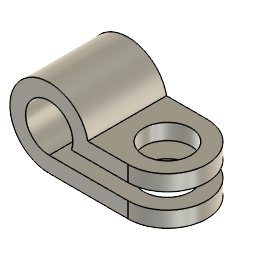
Cable Clip (Autodesk Fusion 360 design; units mm, degrees)
part number: 2025-09-15-17-10-41-254
part number: 2025-09-15-17-13-02-400
Autodesk Fusion 360 part; units mm, degrees
sketch "Sketch1" plane through (0, 0, 0) normal (0, 0, 1) x (1, 0, 0) in component "3mm Cable Clip"
sketch "Sketch2" plane through (0, 0, 0) normal (0, 1, 0) x (1, 0, 0) in component "3mm Cable Clip"
  line L0 (0, 3) -> (15, 3)
  line L1 (0, 0) -> (0, 3) construction
  line L2 (2.8284, 1) -> (15, 1)
  arc A0 (0, 3) -> (2.8284, 1) centre (0, 0) ccw
  dimension "d2" = 6
  dimension "d3" = 15
  dimension "d5" = 2
  constraint coincident L1.start A0.centre
  constraint horizontal L0
  constraint perpendicular L0 L1
  constraint horizontal L2
  constraint vertical L0.end L2.end
  measures "d2" diameter of A0
  measures "d3" distance of L0.start L0.end
  measures "d5" distance of L0 L2
surface "Extrude1" add extruded along (0, 1, 0) between 0 and 10 path "Sketch2" along L0 A0 L2 makes body 1 in component "3mm Cable Clip"
thicken "Thicken1" add thickness 2 3 faces at (-2.5433, 6.6667, 1.5912) (5, 3.3333, -3) (6.8856, 3.3333, -1) separate body on bodies 1 makes body 2 in component "3mm Cable Clip"
fillet "Fillet1" radius 5 4 edges at (15, 10, 0) (15, 10, -4) (15, 0, -4) (15, 0, 0) on bodies 2 in component "3mm Cable Clip"
sketch "Sketch3" plane through (0, 0, 1) normal (0, 0, 1) x (-1, 0, 0) in component "3mm Cable Clip"
  arc A0 (-10, 0) -> (-10, -10) centre (-10, -5) ccw
  line L0 (-10, -10) -> (-4.899, -10)
  line L1 (-4.899, -10) -> (-4.899, 0)
  line L2 (-4.899, 0) -> (-10, 0)
  circle A1 centre (-10, -5) radius 3
  dimension "d12" = 6
  constraint concentric A0 A1
  measures "d12" diameter of A1
extrude "Extrude2" cut sketch "Sketch3" against normal up to surface (6 mm away) contours A1 bodies 2 in component "3mm Cable Clip"
component "3mm Cable Clip" placed x (1, 0, 0) y (0, 1, 0) z (0, 0, 1) at (0, 0, 0)
hidden bodies 1
equation "WireDiameter = 3 mm"
equation "d2 = WireDiameter + 3 mm"
equation "d3 = Width * 1.5"
equation "Width = 10 mm"
equation "d5 = Gap"
equation "Gap = 2 mm"
equation "d7 = Width"
equation "d11 = Width / 2"
